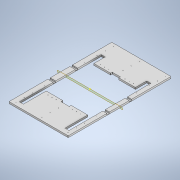
# Autodesk Inventor part: top_part
Saved by Autodesk Inventor 2020 (Build 240168000, 168)
## iProperties
Created: 2019-12-27
Part Number: top_part
Material: Générique
Document SubType Name: Modeling
Designer: damien
Density: 1 g/cm^3
Appearance: Par défaut
Author: damien
Autodesk Inventor part; units mm, degrees
ref_plane "YZ Plane" through (0, 0, 0) normal (1, 0, 0) x (0, 1, 0)
ref_plane "XZ Plane" through (0, 0, 0) normal (0, 1, 0) x (-1, 0, 0)
ref_plane "XY Plane" through (0, 0, 0) normal (0, 0, 1) x (1, 0, 0)
sketch "Esquisse1" plane through (0, 0, 0) normal (0, 1, 0) x (-1, 0, 0)
  line L0 (-360, -625) -> (360, -625)
  line L1 (360, -625) -> (360, 625)
  line L2 (360, 625) -> (-360, 625)
  line L3 (-360, 625) -> (-360, -625)
  line L4 (-360, -625) -> (360, 625) construction
  line L5 (360, -625) -> (-360, 625) construction
  point P0 (0, 0)
  dimension "d0" = 1250
  dimension "d1" = 720
  constraints: 12 end point, 2 midpoint, 2 parallel, 1 horizontal, 1 perpendicular
  measures "d0" distance of L0.end L1.end
  measures "d1" distance of L1.end L2.end
extrude "Extrusion1" add sketch "Esquisse1" along normal blind 21
sketch "Esquisse2" plane through (0, 21, 0) normal (0, 1, 0) x (1, 0, 0)
  line L0 (-295, -565) -> (-295, 430)
  line L1 (-295, 430) -> (-245, 430)
  line L2 (-245, 430) -> (-245, 293)
  line L3 (-245, 293) -> (260, 293)
  line L4 (260, 293) -> (260, 430)
  line L5 (260, 430) -> (310, 430)
  line L6 (310, 430) -> (310, -565)
  line L7 (310, -565) -> (260, -565)
  line L8 (260, -565) -> (260, -287)
  line L9 (260, -287) -> (-245, -287)
  line L10 (-245, -287) -> (-245, -565)
  line L11 (-245, -565) -> (-295, -565)
  line L12 (360, -625) -> (360, 625) projected
  line L13 (360, 0) -> (310, -67.5) construction
  line L14 (-360, 625) -> (-360, -625) projected
  line L15 (-360, -625) -> (360, -625) projected
  line L16 (360, 625) -> (-360, 625) projected
  point P0 (0, 0)
  dimension "d4" = 995
  dimension "d5" = 50
  dimension "d6" = 605
  dimension "d7" = 580
  dimension "d8" = 137
  dimension "d9" = 50
  dimension "d10" = 60
  dimension "d53" = 195
  constraints: 26 end point, 7 perpendicular, 6 point on line, 2 equal length, 2 midpoint, 2 vertical
  measures "d4" distance of L5.end L6.end
  measures "d5" distance of L6.end L7.end
  measures "d6" distance between parallel lines of L0 L6
  measures "d7" distance between parallel lines of L3 L9
  measures "d8" distance of L3.end L4.end
  measures "d9" distance between parallel lines of L12 L6
  measures "d10" distance between parallel lines of L15 L11
  measures "d53" distance between parallel lines of L16 L1
extrude "Extrusion2" cut sketch "Esquisse2" against normal blind 21.1 contours L0 L1 L2 L3 L4 L5 L6 L7 L8 L9 L10 L11
sketch "Esquisse3" plane through (-360, 0, 675) normal (1, 0, 0) x (0, 0, -1)
  line L0 (110, 21) -> (1105, 21) projected
  line L1 (520, 21) -> (550, 21)
  line L2 (550, 21) -> (550, 6)
  line L3 (550, 6) -> (520, 6)
  line L4 (520, 6) -> (520, 21)
  line L5 (50, 0) -> (50, 21) projected
  line L6 (790, 21) -> (820, 21)
  line L7 (820, 21) -> (820, 6)
  line L8 (820, 6) -> (790, 6)
  line L9 (790, 6) -> (790, 21)
  point P0 (675, 0)
  dimension "d13" = 470
  dimension "d14" = 30
  dimension "d15" = 15
  dimension "d16" = 240
  dimension "d17" = 30
  constraints: 16 end point, 4 parallel, 2 horizontal, 2 perpendicular, 2 point on line, 1 collinear
  measures "d13" distance from line of L5 L1.start
  measures "d14" distance of L2.end L3.end
  measures "d15" distance of L1.end L2.end
  measures "d16" distance between parallel lines of L9 L2
  measures "d17" distance of L7.end L8.end
extrude "Extrusion3" cut sketch "Esquisse3" along normal blind 1000
sketch "Esquisse4" plane through (0, 21, 0) normal (0, 1, 0) x (1, 0, 0)
  line L0 (260, 293) -> (-245, 293) projected
  line L1 (-42.5, 293) -> (57.5, 293)
  line L2 (57.5, 293) -> (57.5, 313)
  line L3 (57.5, 313) -> (-42.5, 313)
  line L4 (-42.5, 313) -> (-42.5, 293)
  line L5 (-245, -287) -> (260, -287) projected
  line L6 (-42.5, -287) -> (57.5, -287)
  line L7 (57.5, -287) -> (57.5, -310)
  line L8 (57.5, -310) -> (-42.5, -310)
  line L9 (-42.5, -310) -> (-42.5, -287)
  line L10 (-245, 430) -> (-245, 293) projected
  line L11 (260, 293) -> (260, 430) projected
  point P0 (0, 0)
  dimension "d20" = 23
  dimension "d21" = 100
  dimension "d22" = 202.5
  dimension "d23" = 202.5
  dimension "d50" = 20
  constraints: 16 end point, 4 parallel, 4 point on line, 2 horizontal, 2 perpendicular
  measures "d20" distance of L6.end L7.end
  measures "d21" distance of L2.end L3.end
  measures "d22" distance between parallel lines of L10 L4
  measures "d23" distance between parallel lines of L11 L2
  measures "d50" distance of L1.end L2.end
extrude "Extrusion4" cut sketch "Esquisse4" against normal blind 100
fillet "Congé1" radius 2 8 edges at (57.5, 10.5, -313) (57.5, 10.5, -293) (-42.5, 10.5, -313) (-42.5, 10.5, -293) (-42.5, 10.5, 287) (-42.5, 10.5, 310) (57.5, 10.5, 310) (57.5, 10.5, 287)
sketch "Esquisse5" plane through (0, 21, 0) normal (0, 1, 0) x (1, 0, 0)
  circle A0 centre (7.5, 493) radius 2.25
  circle A1 centre (7.5, 393) radius 2.25
  line L0 (-360, 625) -> (-360, 145) projected
  line L1 (360, -625) -> (360, 625) projected
  circle A2 centre (7.5, 593) radius 2.25
  line L2 (-245, 293) -> (-44.5, 293) projected
  circle A3 centre (326, 593) radius 2.25
  circle A4 centre (326, 493) radius 2.25
  circle A5 centre (326, 393) radius 2.25
  circle A6 centre (-308, 393) radius 2.25
  circle A7 centre (-308, 493) radius 2.25
  circle A8 centre (-308, 593) radius 2.25
  circle A9 centre (-308, 243) radius 2.25
  circle A10 centre (326, 243) radius 2.25
  line L3 (7.5, 393) -> (7.5, 313) construction
  line L4 (55.5, 313) -> (-40.5, 313) projected
  point P0 (0, 0)
  dimension "d29" = 100
  dimension "d30" = 100
  dimension "d32" = 100
  dimension "d35" = 34
  dimension "d36" = 52
  dimension "d51" = 150
  dimension "d52" = 4.5
  constraints: 11 centre point, 11 equal radius, 8 vertical alignment, 7 horizontal alignment, 2 end point, 1 midpoint, 1 vertical
  measures "d29" distance of A0.centre L3.start
  measures "d30" distance of A0.centre A2.centre
  measures "d32" distance from line of L3.start L2
  measures "d35" distance from line of L1 A4.centre
  measures "d36" distance from line of L0 A6.centre
  measures "d51" distance of A9.centre A6.centre
  measures "d52" diameter of A1
extrude "Extrusion5" cut sketch "Esquisse5" against normal blind 100
mirror "Symétrie1" about plane through (0, 0, 0) normal (0, 0, 1) of "Extrusion5"
sketch "Esquisse6" plane through (0, 21, 0) normal (0, 1, 0) x (1, 0, 0)
  circle A0 centre (-192.5, -319) radius 2.25
  line L0 (-245, -565) -> (-245, -287) projected
  line L1 (-245, -319) -> (260, -319) construction
  line L2 (260, -565) -> (260, -287) projected
  line L3 (55.5, -310) -> (-40.5, -310) projected
  circle A1 centre (-142.5, -319) radius 2.25
  circle A2 centre (-92.5, -319) radius 2.25
  line L4 (-40.5, -310) -> (55.5, -310) projected
  line L5 (7.5, -310) -> (7.5, -625) construction
  line L6 (-360, -625) -> (360, -625) projected
  circle A3 centre (207.5, -319) radius 2.25
  circle A4 centre (157.5, -319) radius 2.25
  circle A5 centre (107.5, -319) radius 2.25
  point P0 (0, 0)
  dimension "d37" = 4.5
  dimension "d38" = 9
  dimension "d39" = 52.5
  dimension "d42" = 50
  constraints: 6 centre point, 4 end point, 4 point on line, 3 symmetric about line, 2 horizontal, 2 midpoint, 1 vertical, 7 other
  measures "d37" diameter of A0
  measures "d38" distance between parallel lines of L1 L3
  measures "d39" distance from line of L0 A0.centre
  measures "d42" distance of A0.centre A1.centre
extrude "Extrusion6" cut sketch "Esquisse6" against normal blind 100
mirror "Symétrie3" about plane through (0, 0, 0) normal (0, 0, 1) of "Extrusion6"
sketch "Esquisse7" plane through (0, 21, 0) normal (0, 1, 0) x (1, 0, 0)
  point P0 (0, 0)
fillet "Congé2" radius 5 4 edges at (360, 10.5, -625) (-360, 10.5, -625) (-360, 10.5, 625) (360, 10.5, 625)
ref_plane "Plan de construction1" through (0, 0, 0) normal (0, 0, 1) x (1, 0, 0)
